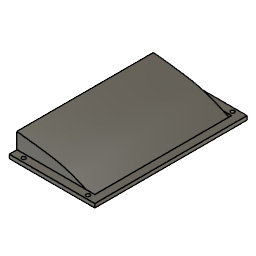
car scoop (Autodesk Fusion 360 design; units mm, degrees)
part number: 2026-04-04-14-47-27-838
Autodesk Fusion 360 part; units mm, degrees
sketch "Sketch1" plane through (0, 0, 0) normal (0, 1, 0) x (1, 0, 0)
  line L0 (0, 0) -> (101.6, 0)
  line L1 (0, 0) -> (0, -25.4)
  spline S0 degree 2 poles (0, -25.4) (61.2882, -18.6006) (101.6, 0) knots 0 0 0 10.537877 10.537877 10.537877 weights 1 2.365825 1
  spline S1 degree 2 poles (0, -20) (59.3611, -12.7) (94.0715, 0) knots 0 0 0 9.650073 9.650073 9.650073 weights 1 3 1
  dimension "d1" = 101.6
  dimension "d2" = 25.4
  constraint coincident L0.start L1.start
  constraint horizontal L0
  constraint perpendicular L0 L1
  constraint coincident L0 S1.end
  constraint coincident L1 S1.start
  measures "d1" distance of L0.start L0.end
  measures "d2" distance of L0.start L1.end
extrude "Extrude1" add sketch "Sketch1" along normal blind 5.08 makes body 1
extrude "Extrude2" add sketch "Sketch1" along normal blind 177.8 separate body contours L0 L1 S0 S1 makes body 2
extrude "Extrude3" add sketch "Sketch1" along normal blind 5.08 from surface at 172.72 separate body makes body 3
sketch "Sketch2" plane through (0, 0, 0) normal (0, 0, 1) x (1, 0, 0)
  line L0 (0.4808, 187.96) -> (111.76, 187.96)
  line L1 (111.76, 187.96) -> (111.76, -10.16)
  line L2 (111.76, -10.16) -> (0.4808, -10.16)
  line L3 (0.4808, -10.16) -> (0.4808, 187.96)
  line L4 (0, 0) -> (0, 177.8)
  line L5 (0, 177.8) -> (101.6, 177.8)
  line L6 (101.6, 0) -> (101.6, 177.8)
  line L7 (0, 0) -> (101.6, 0)
  circle A0 centre (97.9777, -5.1517) radius 2.4447
  line L8 (56.1204, -10.16) -> (56.1204, 187.96) construction
  line L9 (111.76, 88.9) -> (0.4808, 88.9) construction
  circle A1 centre (14.2631, -5.1517) radius 2.4447
  circle A2 centre (97.9777, 182.9517) radius 2.4447
  circle A3 centre (14.2631, 182.9517) radius 2.4447
  dimension "d13" = 10.16
  dimension "d14" = 10.16
  dimension "d15" = 10.16
  dimension "d16" = 4.8895
  constraint horizontal L0
  constraint vertical L1
  constraint horizontal L2
  constraint vertical L3
  constraint midpoint L2 L8.start
  constraint midpoint L0 L8.end
  constraint midpoint L1 L9.start
  constraint midpoint L3 L9.end
  constraint symmetric A0 L8 A1
  constraint symmetric A0 L9 A2
  constraint symmetric L9 A1 A3
  measures "d13" distance of L0 L5
  measures "d14" distance of L1 L6
  measures "d15" distance of L2 L7
  measures "d16" diameter of A0
extrude "Extrude4" add sketch "Sketch2" along normal blind 5.08 separate body contours L0 L1 L2 L3 L5 L6 L7 makes body 4
combine "Combine1" operation add target body 3 tool bodies 4 1 2
